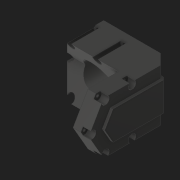
# Autodesk Inventor part: TARM03
Saved by Autodesk Inventor 2017 (Build 210142000, 142)
## iProperties
Created: 2018-10-19
Part Number: TARM03
Material: ABS Plastic
Document SubType Name: Modeling
Designer: Dell
Density: 1.06 g/cm^3
Appearance: Smooth - Black
Author: Dell
Autodesk Inventor part; units mm, degrees
ref_plane "YZ Plane" through (0, 0, 0) normal (1, 0, 0) x (0, 1, 0)
ref_plane "XZ Plane" through (0, 0, 0) normal (0, 1, 0) x (-1, 0, 0)
ref_plane "XY Plane" through (0, 0, 0) normal (0, 0, 1) x (1, 0, 0)
sketch "Sketch41" plane through (0, 0, 0) normal (0, 0, 1) x (1, 0, 0)
  circle A0 centre (0, 0) radius 22.5
  line L0 (-57.5, 0) -> (-28.75, 49.7965)
  line L1 (-28.75, 49.7965) -> (28.75, 49.7965)
  line L2 (28.75, 49.7965) -> (57.5, 0)
  line L3 (57.5, 0) -> (28.75, -49.7965)
  line L4 (28.75, -49.7965) -> (-28.75, -49.7965)
  line L5 (-28.75, -49.7965) -> (-57.5, 0)
  circle A1 centre (51, 0) radius 2.5
  circle A2 centre (25.5, 44.1673) radius 2.5
  circle A3 centre (-25.5, 44.1673) radius 2.5
  circle A4 centre (-51, 0) radius 2.5
  circle A5 centre (-25.5, -44.1673) radius 2.5
  circle A6 centre (25.5, -44.1673) radius 2.5
  line L6 (28.75, 49.7965) -> (100, 49.7965)
  line L7 (100, 49.7965) -> (100, -49.7965)
  line L8 (100, -49.7965) -> (28.75, -49.7965)
  dimension "d169" = 45
  dimension "d170" = 115
  dimension "d171" = 5
  dimension "d172" = 51
  dimension "d175" = 360
  dimension "d179" = 100
  constraints: 18 end point, 7 centre point, 3 coincident, 2 horizontal alignment, 1 collinear, 1 horizontal, 1 perpendicular, 26 other
  measures "d169" diameter of A0
  measures "d170" distance of L0.start L2.end
  measures "d171" diameter of A1
  measures "d172" distance of A1.centre point (0, 0)
  measures "d179" distance from line of L7 point (0, 0)
extrude "Extrusion38" add sketch "Sketch41" along normal blind 30
sketch "Sketch42" plane through (100, -49.7965, 0) normal (1, 0, 0) x (0, 0, -1)
  line L0 (-42.5, 49.7965) -> (-71.25, 0)
  line L1 (-71.25, 0) -> (-128.75, 0)
  line L2 (-128.75, 0) -> (-157.5, 49.7965)
  line L3 (-157.5, 49.7965) -> (-128.75, 99.5929)
  line L4 (-128.75, 99.5929) -> (-71.25, 99.5929)
  line L5 (-71.25, 99.5929) -> (-42.5, 49.7965)
  line L6 (0, 0) -> (0, 99.5929) projected
  circle A0 centre (-100, 49.7965) radius 22.5
  circle A1 centre (-151, 49.7965) radius 2.5
  circle A2 centre (-125.5, 5.6292) radius 2.5
  circle A3 centre (-74.5, 5.6292) radius 2.5
  circle A4 centre (-49, 49.7965) radius 2.5
  circle A5 centre (-74.5, 93.9638) radius 2.5
  circle A6 centre (-125.5, 93.9638) radius 2.5
  line L7 (-71.25, 99.5929) -> (0, 99.5929)
  line L8 (0, 0) -> (0, 49.7965) projected
  line L9 (0, 0) -> (-71.25, 0)
  point P0 (0, 49.7965)
  dimension "d180" = 100
  dimension "d181" = 45
  dimension "d182" = 5
  dimension "d183" = 51
  dimension "d186" = 360
  constraints: 16 end point, 7 centre point, 4 horizontal alignment, 1 coincident, 1 horizontal, 1 midpoint, 1 perpendicular, 26 other
  measures "d180" distance from line of L6 point (-100, 49.796)
  measures "d181" diameter of A0
  measures "d182" diameter of A1
  measures "d183" distance of A1.centre point (-100, 49.796)
extrude "Extrusion39" add sketch "Sketch42" against normal blind 30
sketch "Sketch43" plane through (70, -49.7965, 0) normal (-1, 0, 0) x (0, 0, 1)
  circle A0 centre (100, 49.7965) radius 22.5 construction
  line L0 (158.5, 49.7965) -> (129.25, -0.866) construction
  line L1 (129.25, -0.866) -> (70.75, -0.866)
  line L2 (70.75, -0.866) -> (41.5, 49.7965)
  line L3 (41.5, 49.7965) -> (70.75, 100.4589)
  line L4 (70.75, 100.4589) -> (129.25, 100.4589)
  line L5 (129.25, 100.4589) -> (158.5, 49.7965)
  line L6 (30, 99.5929) -> (30, 49.7965) projected
  line L7 (30, 49.7965) -> (30, 0) projected
  line L8 (30, 99.5929) -> (70.25, 99.5929)
  line L9 (0, 99.5929) -> (128.75, 99.5929) projected
  line L10 (70.25, 99.5929) -> (41.5, 49.7965)
  line L11 (41.5, 49.7965) -> (70.25, 0)
  line L12 (0, 0) -> (128.75, 0) projected
  line L13 (30, 0) -> (70.25, 0)
  point P0 (0, 49.7965)
  dimension "d190" = 117
  constraints: 20 end point, 5 point on line, 2 collinear, 1 coincident, 1 horizontal alignment, 13 other
  measures "d190" distance of L2.end L0.start
extrude "Extrusion40" add sketch "Sketch43" along normal blind 150
sketch "Sketch44" plane through (0, 0, 0) normal (0, 0, -1) x (-1, 0, 0)
  line L0 (28.75, -49.7965) -> (-100, -49.7965) projected
  line L1 (28.75, -49.7965) -> (57.5, 0) projected
  line L2 (57.5, 0) -> (28.75, 49.7965) projected
  line L3 (-100, 49.7965) -> (28.75, 49.7965) projected
  line L4 (-100, -49.7965) -> (-100, 49.7965) construction
  circle A0 centre (-51, 0) radius 2.5 projected
  circle A1 centre (-25.5, 44.1673) radius 2.5 projected
  circle A2 centre (25.5, 44.1673) radius 2.5 projected
  circle A3 centre (51, 0) radius 2.5 projected
  circle A4 centre (25.5, -44.1673) radius 2.5 projected
  circle A5 centre (-25.5, -44.1673) radius 2.5 projected
  circle A6 centre (0, 0) radius 22.5 projected
  line L5 (28.75, 49.7965) -> (57.5, 0) projected
  line L6 (57.5, 0) -> (28.75, -49.7965) projected
  line L7 (28.75, -49.7965) -> (80, -49.7965) projected
  line L8 (80, 49.7965) -> (80, -49.7965) projected
  line L9 (28.75, 49.7965) -> (80, 49.7965) projected
extrude "Extrusion41" cut sketch "Sketch44" against normal through all
sketch "Sketch45" plane through (100, -49.7965, 0) normal (1, 0, 0) x (0, 0, -1)
  circle A0 centre (-100, 49.7965) radius 22.5 projected
  circle A1 centre (-151, 49.7965) radius 2.5 projected
  circle A2 centre (-151, 49.7965) radius 7.5
  circle A3 centre (-125.5, 5.6292) radius 7.5
  circle A4 centre (-74.5, 5.6292) radius 7.5
  circle A5 centre (-49, 49.7965) radius 7.5
  circle A6 centre (-74.5, 93.9638) radius 7.5
  circle A7 centre (-125.5, 93.9638) radius 7.5
  point P0 (0, 49.7965)
  dimension "d195" = 15
  dimension "d198" = 360
  constraints: 6 centre point, 1 coincident, 13 other
  measures "d195" diameter of A2
extrude "Extrusion42" cut sketch "Sketch45" against normal blind 15 contours A0 | A1 | A2 | A3 | A4 | A5 | A6 | A7
ref_plane "Work Plane3" through (0, 0, 15) normal (0, 0, -1) x (-1, 0, 0)
sketch "Sketch46" plane through (0, 0, 15) normal (0, 0, -1) x (-1, 0, 0)
  arc A0 (53.5, 0) -> (48.5, 0) centre (51, 0) ccw projected
  circle A1 centre (51, 0) radius 7.5
  circle A2 centre (25.5, 44.1673) radius 7.5
  circle A3 centre (-25.5, 44.1673) radius 7.5
  circle A4 centre (-51, 0) radius 7.5
  circle A5 centre (-25.5, -44.1673) radius 7.5
  circle A6 centre (25.5, -44.1673) radius 7.5
  point P0 (0, 0)
  dimension "d203" = 15
  dimension "d206" = 360
  constraints: 6 centre point, 1 coincident, 13 other
  measures "d203" diameter of A1
extrude "Extrusion43" cut sketch "Sketch46" against normal through all
sketch "Sketch47" plane through (100, -49.7965, 0) normal (1, 0, 0) x (0, 0, -1)
  line L0 (-29, 41.2965) -> (-17, 41.2965)
  line L1 (-17, 41.2965) -> (-17, 58.2965)
  line L2 (-17, 58.2965) -> (-29, 58.2965)
  line L3 (-29, 58.2965) -> (-29, 41.2965)
  line L4 (0, 0) -> (0, 99.5929) projected
  point P0 (0, 49.7965)
  point P1 (-17, 49.7965)
  point P2 (0, 49.7965)
  dimension "d210" = 17
  dimension "d211" = 17
  dimension "d212" = 12
  constraints: 8 end point, 2 midpoint, 2 parallel, 1 horizontal, 1 horizontal alignment, 1 perpendicular
  measures "d210" distance between parallel lines of L4 L1
  measures "d211" distance of L2.end L0.start
  measures "d212" distance of L1.end L2.end
extrude "Extrusion44" cut sketch "Sketch47" against normal blind 100
chamfer "Chamfer2" distance 20 angle 45 1 edges at (100, 0, 0)
sketch "Sketch48" plane through (100, 0, 151) normal (1, 0, 0) x (0, 0, -1)
  line L0 (122, -8.5) -> (134, -8.5) projected
  line L1 (134, -8.5) -> (49, -8.5)
  line L2 (49, -8.5) -> (49, 8.5)
  line L3 (49, 8.5) -> (134, 8.5)
  line L4 (134, 8.5) -> (134, -8.5)
  point P0 (151, 0)
  point P1 (134, 8.5)
  dimension "d218" = 85
  constraints: 8 end point, 2 parallel, 1 coincident, 1 horizontal, 1 perpendicular
  measures "d218" distance of L2.end L3.end
extrude "Extrusion45" cut sketch "Sketch48" against normal blind 12
sketch "Sketch50" plane through (88, 0, 151) normal (1, 0, 0) x (0, 0, -1)
  arc A0 (71.8327, 8.5) -> (71.8327, -8.5) centre (51, 0) ccw projected
  line L0 (131, 49.7965) -> (131, 8.5) projected
  line L1 (131, -8.5) -> (131, -49.7965) projected
  line L2 (51, 22.5) -> (131, 22.5)
  circle A1 centre (51, 0) radius 22.5 projected
  line L3 (51, -22.5) -> (131, -22.5)
  line L4 (131, 22.5) -> (131, -22.5)
  point P0 (151, 0)
  constraints: 6 end point, 4 point on circle, 3 tangent, 2 point on line, 1 collinear, 1 horizontal, 1 perpendicular
extrude "Extrusion46" cut sketch "Sketch50" along normal through all contours A0 L2 L0 L4 L1 L3 A1
sketch "Sketch51" plane through (88, 0, 151) normal (1, 0, 0) x (0, 0, -1)
  line L0 (131, 49.7965) -> (131, 22.5) projected
  line L1 (131, 27.5) -> (136.6874, 27.5)
  line L2 (136.6874, 27.5) -> (136.6874, -27.5)
  line L3 (136.6874, -27.5) -> (131, -27.5)
  line L4 (131, -27.5) -> (131, 27.5)
  line L5 (51, 22.5) -> (131, 22.5) projected
  point P0 (151, 0)
  point P1 (136.6874, 0)
  dimension "d223" = 5
  constraints: 8 end point, 2 parallel, 1 horizontal, 1 horizontal alignment, 1 midpoint, 1 perpendicular, 1 point on line
  measures "d223" distance between parallel lines of L1 L5
extrude "Extrusion47" add sketch "Sketch51" along normal blind 12
chamfer "Chamfer3" distance 2 angle 45 1 edges at (88, 0, 20)
sketch "Sketch52" plane through (100, 0, 151) normal (1, 0, 0) x (0, 0, -1)
  arc A0 (51, 22.5) -> (51, -22.5) centre (51, 0) ccw projected
  line L0 (19.2457, 0) -> (35.1229, 27.5)
  line L1 (35.1229, 27.5) -> (66.8771, 27.5)
  line L2 (66.8771, 27.5) -> (82.7543, 0) construction
  line L3 (82.7543, 0) -> (66.8771, -27.5) construction
  line L4 (66.8771, -27.5) -> (35.1229, -27.5)
  line L5 (35.1229, -27.5) -> (19.2457, 0)
  line L6 (136.6874, 27.5) -> (131, 27.5) projected
  line L7 (51, 22.5) -> (131, 22.5) projected
  line L8 (131, -22.5) -> (51, -22.5) projected
  line L9 (131, 22.5) -> (131, -22.5) projected
  line L10 (66.8771, 27.5) -> (131, 27.5)
  line L11 (136.6874, -27.5) -> (131, -27.5) projected
  line L12 (66.8771, -27.5) -> (131, -27.5)
  line L13 (136.6874, 27.5) -> (136.6874, -27.5) projected
  line L14 (136.6874, -27.5) -> (136.6874, 27.5)
  point P0 (151, 0)
  point P1 (51, 0)
  constraints: 18 end point, 2 collinear, 2 horizontal alignment, 1 coincident, 1 horizontal, 13 other
extrude "Extrusion48" add sketch "Sketch52" along normal blind 5 contours L7 L9 L8 A0 | L0 L1 L10 L6 L13 L11 L12 L4 L5
chamfer "Chamfer4" distance 5 angle 45 1 edges at (105, 0, 14.3126)
sketch "Sketch53" plane through (88, 0, 151) normal (1, 0, 0) x (0, 0, -1)
  line L0 (134, -8.5) -> (134, 8.5) projected
  line L1 (134, 8.5) -> (122, 8.5) projected
  line L2 (122, 8.5) -> (122, -8.5) projected
  line L3 (122, -8.5) -> (134, -8.5) projected
  line L4 (109.5, 0) -> (109.5, 0) projected
  line L5 (109.5, 0) -> (109.5, 0) projected
  line L6 (151, 22.5) -> (151, -22.5) projected
  line L7 (134, 8.5) -> (134, -8.5) projected
  circle A0 centre (128, 0) radius 10.4043
  point P0 (151, 0)
  point P1 (122, 0)
  point P2 (128, 8.5)
  constraints: 2 midpoint, 1 horizontal alignment, 1 vertical alignment, 3 other
extrude "Extrusion49" cut sketch "Sketch53" against normal blind 75 and the other way blind 3
body "Solid2"
